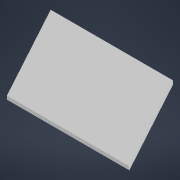
# Autodesk Inventor part: TorraumSchrägeObenNEU
Saved by Autodesk Inventor 2021.4 (Build 254397000, 397)
## iProperties
Created: 2022-02-22
Part Number: TorraumSchrägeObenNEU
Material: Generisch
Document SubType Name: Modeling
Designer: valen
Density: 1 g/cm^3
Appearance: Vorgabe
Author: valen
Autodesk Inventor part; units mm, degrees
ref_plane "YZ Plane" through (0, 0, 0) normal (1, 0, 0) x (0, 1, 0)
ref_plane "XZ Plane" through (0, 0, 0) normal (0, 1, 0) x (-1, 0, 0)
ref_plane "XY Plane" through (0, 0, 0) normal (0, 0, 1) x (1, 0, 0)
sketch "Skizze1" plane through (0, 0, 0) normal (1, 0, 0) x (0, 1, 0)
  line L0 (0, 0) -> (97, 0) construction
  line L1 (-6.2482, 0) -> (-6.2482, -80)
  line L2 (-6.2482, -80) -> (89.7518, -80)
  line L3 (89.7518, -80) -> (-6.2482, 0)
  line L4 (89.7518, -80) -> (96, -80)
  line L5 (96, -80) -> (0, 0)
  line L6 (-6.2482, 0) -> (0, 0)
  dimension "d7" = 80
  dimension "d8" = 96
  dimension "d12" = 4
  constraints: 14 end point, 3 horizontal, 2 parallel, 1 vertical
  measures "d7" distance of L1.start L1.end
  measures "d8" distance of L1.end L2.end
  measures "d12" distance between parallel lines of L3 L5
extrude "Extrusion2" add sketch "Skizze1" along normal blind 224 contours L6 L5 L4 L3
